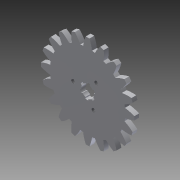
# Autodesk Inventor part: Small Spur Gear
Saved by Autodesk Inventor 2014 SP1 (Build 180222100, 222)
## iProperties
Created: 2012-03-30
Part Number: Small Spur Gear
Material: Aluminum-6061
Document SubType Name: Modeling
Designer: Moses
Mass: 162.936 g
Surface Area: 240.137 cm^2
Volume: 60.124 cm^3
Density: 2.71 g/cm^3
Appearance: Aluminum - Flat
Author: Moses
Autodesk Inventor part; units mm, degrees
ref_plane "YZ Plane" through (0, 0, 0) normal (1, 0, 0) x (0, 1, 0)
ref_plane "XZ Plane" through (0, 0, 0) normal (0, 1, 0) x (-1, 0, 0)
ref_plane "XY Plane" through (0, 0, 0) normal (0, 0, 1) x (1, 0, 0)
sketch "Sketch1" plane through (0, 0, 0) normal (0, 0, 1) x (1, 0, 0)
  arc A0 (-21.2148, 57.5054) -> (-20.6771, 44.8522) centre (21.9016, 52.9996) ccw
  arc A1 (-20.6771, 44.8522) -> (-24.1325, 43.0916) centre (0, 0) ccw
  arc A2 (-24.1325, 43.0916) -> (-34.053, 50.964) centre (-55.7511, 13.4336) ccw
  arc A3 (-34.053, 50.964) -> (-37.9467, 48.1351) centre (0, 0) ccw
  arc A4 (-37.9467, 48.1351) -> (-33.5252, 36.2674) centre (4.4519, 57.1736) ccw
  arc A5 (-33.5252, 36.2674) -> (-36.2674, 33.5252) centre (0, 0) ccw
  arc A6 (-36.2674, 33.5252) -> (-48.1351, 37.9467) centre (-57.1736, -4.4519) ccw
  arc A7 (-48.1351, 37.9467) -> (-50.964, 34.053) centre (0, 0) ccw
  arc A8 (-50.964, 34.053) -> (-43.0916, 24.1325) centre (-13.4336, 55.7511) ccw
  arc A9 (-43.0916, 24.1325) -> (-44.8522, 20.6771) centre (0, 0) ccw
  arc A10 (-44.8522, 20.6771) -> (-57.5054, 21.2148) centre (-52.9996, -21.9016) ccw
  arc A11 (-57.5054, 21.2148) -> (-58.9926, 16.6376) centre (0, 0) ccw
  arc A12 (-58.9926, 16.6376) -> (-48.4399, 9.6353) centre (-30.0041, 48.8712) ccw
  arc A13 (-48.4399, 9.6353) -> (-49.0465, 5.805) centre (0, 0) ccw
  arc A14 (-49.0465, 5.805) -> (-61.2466, 2.4064) centre (-43.6377, -37.2075) ccw
  arc A15 (-61.2466, 2.4064) -> (-61.2466, -2.4064) centre (0, 0) ccw
  arc A16 (-61.2466, -2.4064) -> (-49.0465, -5.805) centre (-43.6377, 37.2075) ccw
  arc A17 (-49.0465, -5.805) -> (-48.4399, -9.6353) centre (0, 0) ccw
  arc A18 (-48.4399, -9.6353) -> (-58.9926, -16.6376) centre (-30.0041, -48.8712) ccw
  arc A19 (-58.9926, -16.6376) -> (-57.5054, -21.2148) centre (0, 0) ccw
  arc A20 (-57.5054, -21.2148) -> (-44.8522, -20.6771) centre (-52.9996, 21.9016) ccw
  arc A21 (-44.8522, -20.6771) -> (-43.0916, -24.1325) centre (0, 0) ccw
  arc A22 (-43.0916, -24.1325) -> (-50.964, -34.053) centre (-13.4336, -55.7511) ccw
  arc A23 (-50.964, -34.053) -> (-48.1351, -37.9467) centre (0, 0) ccw
  arc A24 (-48.1351, -37.9467) -> (-36.2674, -33.5252) centre (-57.1736, 4.4519) ccw
  arc A25 (-36.2674, -33.5252) -> (-33.5252, -36.2674) centre (0, 0) ccw
  arc A26 (-33.5252, -36.2674) -> (-37.9467, -48.1351) centre (4.4519, -57.1736) ccw
  arc A27 (-37.9467, -48.1351) -> (-34.053, -50.964) centre (0, 0) ccw
  arc A28 (-34.053, -50.964) -> (-24.1325, -43.0916) centre (-55.7511, -13.4336) ccw
  arc A29 (-24.1325, -43.0916) -> (-20.6771, -44.8522) centre (0, 0) ccw
  arc A30 (-20.6771, -44.8522) -> (-21.2148, -57.5054) centre (21.9016, -52.9996) ccw
  arc A31 (-21.2148, -57.5054) -> (-16.6376, -58.9926) centre (0, 0) ccw
  arc A32 (-16.6376, -58.9926) -> (-9.6353, -48.4399) centre (-48.8712, -30.0041) ccw
  arc A33 (-9.6353, -48.4399) -> (-5.805, -49.0465) centre (0, 0) ccw
  arc A34 (-5.805, -49.0465) -> (-2.4064, -61.2466) centre (37.2075, -43.6377) ccw
  arc A35 (-2.4064, -61.2466) -> (2.4064, -61.2466) centre (0, 0) ccw
  arc A36 (2.4064, -61.2466) -> (5.805, -49.0465) centre (-37.2075, -43.6377) ccw
  arc A37 (5.805, -49.0465) -> (9.6353, -48.4399) centre (0, 0) ccw
  arc A38 (9.6353, -48.4399) -> (16.6376, -58.9926) centre (48.8712, -30.0041) ccw
  arc A39 (16.6376, -58.9926) -> (21.2148, -57.5054) centre (0, 0) ccw
  arc A40 (21.2148, -57.5054) -> (20.6771, -44.8522) centre (-21.9016, -52.9996) ccw
  arc A41 (20.6771, -44.8522) -> (24.1325, -43.0916) centre (0, 0) ccw
  arc A42 (24.1325, -43.0916) -> (34.053, -50.964) centre (55.7511, -13.4336) ccw
  arc A43 (34.053, -50.964) -> (37.9467, -48.1351) centre (0, 0) ccw
  arc A44 (37.9467, -48.1351) -> (33.5252, -36.2674) centre (-4.4519, -57.1736) ccw
  arc A45 (33.5252, -36.2674) -> (36.2674, -33.5252) centre (0, 0) ccw
  arc A46 (36.2674, -33.5252) -> (48.1351, -37.9467) centre (57.1736, 4.4519) ccw
  arc A47 (48.1351, -37.9467) -> (50.964, -34.053) centre (0, 0) ccw
  arc A48 (50.964, -34.053) -> (43.0916, -24.1325) centre (13.4336, -55.7511) ccw
  arc A49 (43.0916, -24.1325) -> (44.8522, -20.6771) centre (0, 0) ccw
  arc A50 (44.8522, -20.6771) -> (57.5054, -21.2148) centre (52.9996, 21.9016) ccw
  arc A51 (57.5054, -21.2148) -> (58.9926, -16.6376) centre (0, 0) ccw
  arc A52 (58.9926, -16.6376) -> (48.4399, -9.6353) centre (30.0041, -48.8712) ccw
  arc A53 (48.4399, -9.6353) -> (49.0465, -5.805) centre (0, 0) ccw
  arc A54 (49.0465, -5.805) -> (61.2466, -2.4064) centre (43.6377, 37.2075) ccw
  arc A55 (61.2466, -2.4064) -> (61.2466, 2.4064) centre (0, 0) ccw
  arc A56 (61.2466, 2.4064) -> (49.0465, 5.805) centre (43.6377, -37.2075) ccw
  arc A57 (49.0465, 5.805) -> (48.4399, 9.6353) centre (0, 0) ccw
  arc A58 (48.4399, 9.6353) -> (58.9926, 16.6376) centre (30.0041, 48.8712) ccw
  arc A59 (58.9926, 16.6376) -> (57.5054, 21.2148) centre (0, 0) ccw
  arc A60 (57.5054, 21.2148) -> (44.8522, 20.6771) centre (52.9996, -21.9016) ccw
  arc A61 (44.8522, 20.6771) -> (43.0916, 24.1325) centre (0, 0) ccw
  arc A62 (43.0916, 24.1325) -> (50.964, 34.053) centre (13.4336, 55.7511) ccw
  arc A63 (50.964, 34.053) -> (48.1351, 37.9467) centre (0, 0) ccw
  arc A64 (48.1351, 37.9467) -> (36.2674, 33.5252) centre (57.1736, -4.4519) ccw
  arc A65 (36.2674, 33.5252) -> (33.5252, 36.2674) centre (0, 0) ccw
  arc A66 (33.5252, 36.2674) -> (37.9467, 48.1351) centre (-4.4519, 57.1736) ccw
  arc A67 (37.9467, 48.1351) -> (34.053, 50.964) centre (0, 0) ccw
  arc A68 (34.053, 50.964) -> (24.1325, 43.0916) centre (55.7511, 13.4336) ccw
  arc A69 (24.1325, 43.0916) -> (20.6771, 44.8522) centre (0, 0) ccw
  arc A70 (20.6771, 44.8522) -> (21.2148, 57.5054) centre (-21.9016, 52.9996) ccw
  arc A71 (21.2148, 57.5054) -> (16.6376, 58.9926) centre (0, 0) ccw
  arc A72 (16.6376, 58.9926) -> (9.6353, 48.4399) centre (48.8712, 30.0041) ccw
  arc A73 (9.6353, 48.4399) -> (5.805, 49.0465) centre (0, 0) ccw
  arc A74 (5.805, 49.0465) -> (2.4064, 61.2466) centre (-37.2075, 43.6377) ccw
  arc A75 (2.4064, 61.2466) -> (-2.4064, 61.2466) centre (0, 0) ccw
  arc A76 (-2.4064, 61.2466) -> (-5.805, 49.0465) centre (37.2075, 43.6377) ccw
  arc A77 (-5.805, 49.0465) -> (-9.6353, 48.4399) centre (0, 0) ccw
  arc A78 (-9.6353, 48.4399) -> (-16.6376, 58.9926) centre (-48.8712, 30.0041) ccw
  arc A79 (-16.6376, 58.9926) -> (-21.2148, 57.5054) centre (0, 0) ccw
  point P0 (0, 0)
  constraints: 160 point on circle, 80 centre point
extrude "Extrusion1" add sketch "Sketch1" along normal blind 6.35
sketch "Sketch2" plane through (0, 0, 0) normal (0, 0, -1) x (-1, 0, 0)
  arc A0 (-1.0922, -8.1269) -> (2.8824, -7.6767) centre (0, 0) ccw projected
  arc A1 (2.8824, -7.6767) -> (6.492, -5.0093) centre (0, 0) ccw projected
  arc A2 (6.492, -5.0093) -> (8.0894, -1.3421) centre (0, 0) ccw projected
  arc A3 (8.0894, -1.3421) -> (7.5842, 3.1176) centre (0, 0) ccw projected
  arc A4 (7.5842, 3.1176) -> (5.207, 6.3346) centre (0, 0) ccw projected
  arc A5 (5.207, 6.3346) -> (1.0922, 8.1269) centre (0, 0) ccw projected
  arc A6 (1.0922, 8.1269) -> (-2.8824, 7.6767) centre (0, 0) ccw projected
  arc A7 (-2.8824, 7.6767) -> (-6.492, 5.0093) centre (0, 0) ccw projected
  arc A8 (-6.492, 5.0093) -> (-8.0894, 1.3421) centre (0, 0) ccw projected
  arc A9 (-8.0894, 1.3421) -> (-7.5842, -3.1176) centre (0, 0) ccw projected
  arc A10 (-7.5842, -3.1176) -> (-5.207, -6.3346) centre (0, 0) ccw projected
  arc A11 (-5.207, -6.3346) -> (-1.0922, -8.1269) centre (0, 0) ccw projected
  line L0 (1.0922, 8.1269) -> (0.8902, 9.9101) projected
  arc A12 (0.8902, 9.9101) -> (-3.0844, 9.4599) centre (0, 0) ccw projected
  line L1 (-3.0844, 9.4599) -> (-2.8824, 7.6767) projected
  line L2 (-6.492, 5.0093) -> (-8.1373, 5.726) projected
  arc A13 (-8.1373, 5.726) -> (-9.7347, 2.0588) centre (0, 0) ccw projected
  line L3 (-9.7347, 2.0588) -> (-8.0894, 1.3421) projected
  line L4 (-7.5842, -3.1176) -> (-9.0275, -4.1841) projected
  arc A14 (-9.0275, -4.1841) -> (-6.6503, -7.4011) centre (0, 0) ccw projected
  line L5 (-6.6503, -7.4011) -> (-5.207, -6.3346) projected
  line L6 (-1.0922, -8.1269) -> (-0.8902, -9.9101) projected
  arc A15 (-0.8902, -9.9101) -> (3.0844, -9.4599) centre (0, 0) ccw projected
  line L7 (3.0844, -9.4599) -> (2.8824, -7.6767) projected
  line L8 (6.492, -5.0093) -> (8.1373, -5.726) projected
  arc A16 (8.1373, -5.726) -> (9.7347, -2.0588) centre (0, 0) ccw projected
  line L9 (9.7347, -2.0588) -> (8.0894, -1.3421) projected
  line L10 (7.5842, 3.1176) -> (9.0275, 4.1841) projected
  arc A17 (9.0275, 4.1841) -> (6.6503, 7.4011) centre (0, 0) ccw projected
  line L11 (6.6503, 7.4011) -> (5.207, 6.3346) projected
extrude "Extrusion2" cut sketch "Sketch2" against normal blind 25.4
sketch "Sketch3" plane through (0, 0, 0) normal (0, 0, -1) x (-1, 0, 0)
  circle A0 centre (-11.3215, 15.3208) radius 2.3495 projected
  circle A1 centre (18.9289, 2.1443) radius 2.3495 projected
  circle A2 centre (-7.6075, -17.4651) radius 2.3495 projected
extrude "Extrusion3" cut sketch "Sketch3" against normal blind 25.4
thread "Thread1" size "10-24 UNC" class "2B" standard "ANSI Unified Screw Threads" full length
thread "Thread2" size "10-24 UNC" class "2B" standard "ANSI Unified Screw Threads" full length
thread "Thread3" size "10-24 UNC" class "2B" standard "ANSI Unified Screw Threads" full length
body "Solid1"
